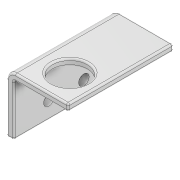
# Autodesk Inventor part: Guia para cable de motor
Saved by Autodesk Inventor 2020 (Build 240168000, 168)
## iProperties
Created: 2020-09-03
Part Number: Guia para cable de motor
Material: Aluminio 1100-H14
Document SubType Name: Modeling
Designer: Pipi
Density: 2.7 g/cm^3
Appearance: Satinado
Author: Pipi
Autodesk Inventor part; units mm, degrees
ref_plane "YZ Plane" through (0, 0, 0) normal (1, 0, 0) x (0, 1, 0)
ref_plane "XZ Plane" through (0, 0, 0) normal (0, 1, 0) x (-1, 0, 0)
ref_plane "XY Plane" through (0, 0, 0) normal (0, 0, 1) x (1, 0, 0)
sketch "Boceto2" plane through (0, 0, 0) normal (0, 1, 0) x (-1, 0, 0)
  line L0 (12.9565, 32.7253) -> (12.9565, 2.7253)
  line L1 (12.9565, 2.7253) -> (-17.0435, 2.7253)
  line L2 (-17.0435, 2.7253) -> (-17.0435, 32.7253)
  line L3 (-17.0435, 32.7253) -> (12.9565, 32.7253)
  line L4 (-2.0435, 2.7253) -> (-2.0435, 32.7253)
  line L5 (12.9565, 32.7253) -> (12.9565, 27.7253)
  line L6 (12.9565, 2.7253) -> (12.9565, 7.7253)
  circle A0 centre (7.9565, 22.7253) radius 1.5
  circle A1 centre (7.9565, 12.7253) radius 1.5
  circle A2 centre (-9.5435, 24.7253) radius 5
  line L7 (-2.0435, 32.7253) -> (-9.5435, 32.7253)
  point P0 (0, 0)
  dimension "d0" = 30
  dimension "d1" = 30
  dimension "d5" = 3
  dimension "d6" = 3
  dimension "d14" = 10
  dimension "d15" = 7.5
  dimension "d17" = 8
  dimension "d19" = 10
  dimension "d20" = 10
  constraints: 16 end point, 3 centre point, 3 perpendicular, 3 point on line, 2 midpoint, 1 vertical
  measures "d0" distance of L0.start L0.end
  measures "d1" distance of L0.end L1.end
  measures "d5" diameter of A0
  measures "d6" diameter of A1
  measures "d14" diameter of A2
  measures "d15" distance of L4.end L7.end
  measures "d17" distance of L7.end A2.centre
  measures "d19" distance of A0.centre A1.centre
  measures "d20" distance from line of L3 A0.centre
extrude "Extrusión1" add sketch "Boceto2" along normal blind 2 contours L0 L1 L4 L3
extrude "Extrusión2" add sketch "Boceto2" along normal blind 2 contours L4 L1 L2 L3
bend part "Pieza de plegado1" radius 0.5 angle 90 line through (2.0435, 0, 2.7253) along (0, 0, 1) centre toward (0, -1, 0) moving side (-1, 0, 0) both sides no
fillet "Empalme1" radius 0.5 20 edges at (1.69, -0.1464, 2.7253) (1.5435, -7.6073, 2.7253) (9.5435, 0, 2.7253) (1.69, -0.1464, 32.7253) (1.5435, -7.6073, 32.7253) (9.5435, 0, 32.7253) (0.2758, 1.2678, 2.7253) (-0.4565, -7.6073, 2.7253) (9.5435, 2, 2.7253) (0.5435, -14.7146, 2.7253) (1.5435, -14.7146, 17.7253) (17.0435, 0, 17.7253) (17.0435, 1, 2.7253) (17.0435, 2, 17.7253) (17.0435, 1, 32.7253) (0.2758, 1.2678, 32.7253) (-0.4565, -7.6073, 32.7253) (9.5435, 2, 32.7253) (0.5435, -14.7146, 32.7253) (-0.4565, -14.7146, 17.7253)
fillet "Empalme2" radius 0.5 2 edges at (14.5435, 0, 24.7253) (14.5435, 2, 24.7253)
